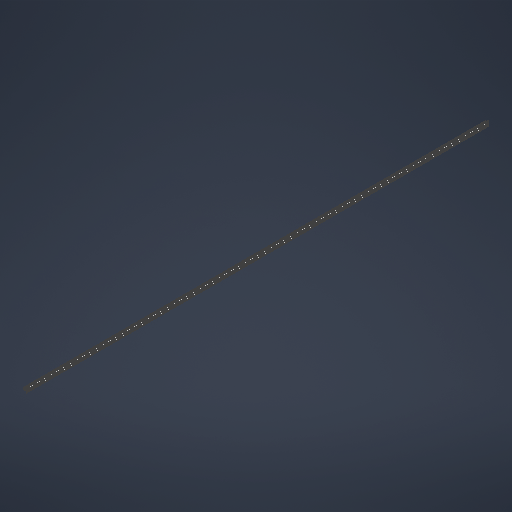
# Autodesk Inventor part: PLANTILLA SP40-04A TRAVESAÑO CENTRAL
Saved by Autodesk Inventor 2025 (Build 290162000, 162)
## iProperties
Created: 2026-01-20
Part Number: PLANTILLA SP40-04A TRAVESAÑO CENTRAL
Material: Aluminio
Document SubType Name: Modeling
Designer: ROLANDO
Density: 2.7 g/cm^3
Appearance: Satinado
Author: ROLANDO
Autodesk Inventor part; units mm, degrees
ref_plane "YZ Plane" through (0, 0, 0) normal (1, 0, 0) x (0, 1, 0)
ref_plane "XZ Plane" through (0, 0, 0) normal (0, 1, 0) x (-1, 0, 0)
ref_plane "XY Plane" through (0, 0, 0) normal (0, 0, 1) x (1, 0, 0)
sketch "Boceto1" plane through (0, 0, 0) normal (0, 0, 1) x (1, 0, 0)
  line L0 (-1.1139, -2.6665) -> (15.7105, -2.6665)
  line L1 (16.2861, -3.2421) -> (16.2861, -16.3665)
  line L2 (16.2861, -16.3665) -> (12.4861, -16.3665)
  line L3 (12.4861, -16.3665) -> (12.4861, -18.0065)
  line L4 (13.1802, -19.0165) -> (13.8861, -19.0165)
  line L5 (13.8861, -19.0165) -> (13.8861, -17.7665)
  line L6 (13.8861, -17.7665) -> (16.2861, -17.7665)
  line L7 (16.2861, -17.7665) -> (16.2861, -24.2665)
  line L8 (16.2861, -24.2665) -> (13.8861, -24.2665)
  line L9 (13.8861, -24.2665) -> (13.8861, -23.0165)
  line L10 (13.8861, -23.0165) -> (13.1802, -23.0165)
  line L11 (12.4861, -24.0265) -> (12.4861, -25.6665)
  line L12 (12.4861, -25.6665) -> (17.6861, -25.6665)
  line L13 (17.6861, -25.6665) -> (17.6861, 4.4835)
  line L14 (16.2861, -0.6909) -> (16.2861, 9.7335)
  line L15 (7.3361, 2.6189) -> (7.3361, -2.6665) construction
  arc A0 (6.2361, 3.2888) -> (8.4361, 3.2888) centre (7.3361, 1.3835) ccw
  line L16 (4.9491, 1.1335) -> (5.1503, 1.1335)
  line L17 (4.9491, 1.6335) -> (5.1503, 1.6335)
  line L18 (10.9772, -1.2665) -> (15.7105, -1.2665)
  line L19 (9.723, 1.1335) -> (9.5218, 1.1335)
  line L20 (9.723, 1.6335) -> (9.5218, 1.6335)
  line L21 (7.5861, -1.0034) -> (7.5861, -0.8022)
  line L22 (7.0861, -1.0034) -> (7.0861, -0.8022)
  arc A1 (7.0861, -1.0034) -> (7.5861, -1.0034) centre (7.3361, 1.3835) ccw
  arc A2 (9.723, 1.1335) -> (9.723, 1.6335) centre (7.3361, 1.3835) ccw
  arc A3 (4.9491, 1.6335) -> (4.9491, 1.1335) centre (7.3361, 1.3835) ccw
  circle A4 centre (7.3361, 1.3835) radius 2.4 construction
  line L23 (6.2361, 4.8271) -> (6.2361, 3.2888)
  line L24 (8.4361, 4.8271) -> (8.4361, 3.2888)
  arc A5 (10.4771, -0.406) -> (8.4361, 4.8271) centre (7.3361, 1.3835) ccw
  arc A6 (6.2361, 4.8271) -> (4.2085, -0.4294) centre (7.3361, 1.3835) ccw
  line L25 (12.4861, -18.0065) -> (13.1802, -19.0165)
  line L26 (12.4861, -24.0265) -> (13.1802, -23.0165)
  arc A7 (15.7105, -1.2665) -> (16.2861, -0.6909) centre (15.7105, -0.6909) ccw
  arc A8 (16.2861, -3.2421) -> (15.7105, -2.6665) centre (15.7105, -3.2421) ccw
  arc A9 (3.8851, -1.2665) -> (4.2085, -0.4294) centre (3.7105, -0.718) ccw
  arc A10 (10.4771, -0.406) -> (10.9772, -1.2665) centre (10.9772, -0.6909) ccw
  line L27 (-26.537, 4.4835) -> (21.9694, 4.4835) construction
  line L28 (-1.6139, -3.1665) -> (-1.6139, -7.0665)
  line L29 (-1.6139, -7.0665) -> (-4.0139, -7.0665)
  line L30 (-5.0139, -5.6665) -> (-3.5139, -5.6665)
  line L31 (-3.0139, -5.1665) -> (-3.0139, -3.1665)
  line L32 (-3.5139, -2.6665) -> (-20.7139, -2.6665)
  line L33 (-21.2139, -3.1665) -> (-21.2139, -5.1665)
  line L34 (-20.7139, -5.6665) -> (-19.2139, -5.6665)
  line L35 (-20.2139, -7.0665) -> (-22.6139, -7.0665)
  line L36 (3.8851, -1.2665) -> (-20.7139, -1.2665)
  line L37 (-21.2139, -0.7665) -> (-21.2139, 4.4835)
  line L38 (-22.6139, -7.0665) -> (-22.6139, 4.4835)
  line L39 (-19.2139, -5.6665) -> (-19.2139, -6.2653)
  line L40 (-19.2139, -6.2653) -> (-20.2139, -7.0665)
  line L41 (-5.0139, -5.6665) -> (-5.0139, -6.2653)
  line L42 (-5.0139, -6.2653) -> (-4.0139, -7.0665)
  line L43 (4.3997, 1.3835) -> (10.1666, 1.3835) construction
  arc A11 (-1.1139, -2.6665) -> (-1.6139, -3.1665) centre (-1.1139, -3.1665) ccw
  arc A12 (-3.0139, -3.1665) -> (-3.5139, -2.6665) centre (-3.5139, -3.1665) ccw
  arc A13 (-3.5139, -5.6665) -> (-3.0139, -5.1665) centre (-3.5139, -5.1665) ccw
  arc A14 (-20.7139, -2.6665) -> (-21.2139, -3.1665) centre (-20.7139, -3.1665) ccw
  arc A15 (-21.2139, -5.1665) -> (-20.7139, -5.6665) centre (-20.7139, -5.1665) ccw
  arc A16 (-21.2139, -0.7665) -> (-20.7139, -1.2665) centre (-20.7139, -0.7665) ccw
  line L44 (-1.1139, 11.6335) -> (15.7105, 11.6335)
  line L45 (16.2861, 12.2091) -> (16.2861, 25.3335)
  line L46 (16.2861, 25.3335) -> (12.4861, 25.3335)
  line L47 (12.4861, 25.3335) -> (12.4861, 26.9735)
  line L48 (13.1802, 27.9835) -> (13.8861, 27.9835)
  line L49 (13.8861, 27.9835) -> (13.8861, 26.7335)
  line L50 (13.8861, 26.7335) -> (16.2861, 26.7335)
  line L51 (16.2861, 26.7335) -> (16.2861, 33.2335)
  line L52 (16.2861, 33.2335) -> (13.8861, 33.2335)
  line L53 (13.8861, 33.2335) -> (13.8861, 31.9835)
  line L54 (13.8861, 31.9835) -> (13.1802, 31.9835)
  line L55 (12.4861, 32.9935) -> (12.4861, 34.6335)
  line L56 (12.4861, 34.6335) -> (17.6861, 34.6335)
  line L57 (17.6861, 34.6335) -> (17.6861, 4.4835)
  line L58 (12.4861, 26.9735) -> (13.1802, 27.9835)
  line L59 (12.4861, 32.9935) -> (13.1802, 31.9835)
  arc A17 (15.7105, 11.6335) -> (16.2861, 12.2091) centre (15.7105, 12.2091) ccw
  line L60 (-1.6139, 12.1335) -> (-1.6139, 16.0335)
  line L61 (-1.6139, 16.0335) -> (-4.0139, 16.0335)
  line L62 (-5.0139, 14.6335) -> (-3.5139, 14.6335)
  line L63 (-3.0139, 14.1335) -> (-3.0139, 12.1335)
  line L64 (-3.5139, 11.6335) -> (-20.7139, 11.6335)
  line L65 (-21.2139, 12.1335) -> (-21.2139, 14.1335)
  line L66 (-20.7139, 14.6335) -> (-19.2139, 14.6335)
  line L67 (-20.2139, 16.0335) -> (-22.6139, 16.0335)
  line L68 (15.7861, 10.2335) -> (-20.7139, 10.2335)
  line L69 (-21.2139, 9.7335) -> (-21.2139, 4.4835)
  line L70 (-22.6139, 16.0335) -> (-22.6139, 4.4835)
  line L71 (-19.2139, 14.6335) -> (-19.2139, 15.2323)
  line L72 (-19.2139, 15.2323) -> (-20.2139, 16.0335)
  line L73 (-5.0139, 14.6335) -> (-5.0139, 15.2323)
  line L74 (-5.0139, 15.2323) -> (-4.0139, 16.0335)
  arc A18 (-1.6139, 12.1335) -> (-1.1139, 11.6335) centre (-1.1139, 12.1335) ccw
  arc A19 (-3.5139, 11.6335) -> (-3.0139, 12.1335) centre (-3.5139, 12.1335) ccw
  arc A20 (-3.0139, 14.1335) -> (-3.5139, 14.6335) centre (-3.5139, 14.1335) ccw
  arc A21 (-21.2139, 12.1335) -> (-20.7139, 11.6335) centre (-20.7139, 12.1335) ccw
  arc A22 (-20.7139, 14.6335) -> (-21.2139, 14.1335) centre (-20.7139, 14.1335) ccw
  arc A23 (-20.7139, 10.2335) -> (-21.2139, 9.7335) centre (-20.7139, 9.7335) ccw
  arc A24 (16.2861, 9.7335) -> (15.7861, 10.2335) centre (15.7861, 9.7335) ccw
  point P0 (4.8546, -1.2453)
  point P1 (9.7949, -1.2665)
  point P2 (7.2983, -2.6665)
  point P3 (16.2861, -21.0165)
  point P4 (5.0497, 1.6335)
  point P5 (9.6224, 1.6335)
  point P6 (16.2861, 29.9835)
  dimension "d4" = 1.4
  dimension "d5" = 1.4
  dimension "d6" = 1.4
  dimension "d7" = 1.4
  dimension "d8" = 1.4
  dimension "d9" = 1.4
  dimension "d12" = 4.4
  dimension "d19" = 0.5
  dimension "d22" = 4.05
  dimension "d26" = 0.5
  dimension "d30" = 0.5
  dimension "d32" = 4.8
  dimension "d35" = 1.1
  dimension "d36" = 2.2
  dimension "d37" = 1.415
  dimension "d38" = 1.415
  dimension "d39" = 0.2
  dimension "d40" = 0.2
  dimension "d43" = 23
  dimension "d44" = 4
  dimension "d45" = 9.3
  dimension "d46" = 6.5
  dimension "d50" = 5.2
  dimension "d53" = 0.2
  dimension "d55" = 0.2
  dimension "d56" = 0.25
  dimension "d57" = 0.2
  dimension "d58" = 1.4
  dimension "d66" = 2
  dimension "d67" = 2
  dimension "d68" = 2.4
  dimension "d69" = 3.01
  dimension "d70" = 6.02
  dimension "d71" = 34.5
  dimension "d72" = 111
  dimension "d74" = 0.7058
  dimension "d75" = 0.7058
  dimension "d90" = 30.15
  dimension "d91" = 1.4
  dimension "d92" = 1.4
  dimension "d93" = 1.4
  dimension "d94" = 1.4
  dimension "d96" = 3
  dimension "d97" = 14.2
  dimension "d98" = 18.2
  dimension "d99" = 21
  dimension "d100" = 40.3
  dimension "d101" = 10.35
  dimension "d102" = 0.25
  dimension "d103" = 0.25
  dimension "d105" = 3.4
  dimension "d106" = 3.4
  dimension "d107" = 1
  dimension "d108" = 38.7
  dimension "d109" = 38.7
  dimension "d118" = 0.5
  dimension "d143" = 0.5
  dimension "d144" = 60.3
  dimension "d145" = 14.3
  dimension "d146" = 23.1
  dimension "d147" = 11.5
  dimension "d148" = 0.5756
  dimension "d149" = 1.4
  dimension "d150" = 4.2833
  constraints: 150 end point, 56 point on circle, 44 symmetric about line, 25 centre point, 21 tangent, 17 perpendicular, 13 point on line, 8 equal radius, 7 parallel, 6 collinear, 6 horizontal, 6 vertical, 4 midpoint, 3 coincident, 2 equal length, 7 other
  measures "d4" distance between parallel lines of L13 L1
  measures "d5" distance between parallel lines of L13 L7
  measures "d6" distance between parallel lines of L12 L8
  measures "d7" distance between parallel lines of L2 L6
  measures "d8" distance between parallel lines of L3 L5
  measures "d9" distance between parallel lines of L11 L9
  measures "d12" diameter of A0
  measures "d19" distance between parallel lines of L16 L17
  measures "d22" distance from line of A5.centre L0
  measures "d26" distance between parallel lines of L19 L20
  measures "d30" distance between parallel lines of L22 L21
  measures "d32" diameter of A4
  measures "d35" distance between parallel lines of L15 L23
  measures "d36" distance between parallel lines of L24 L23
  measures "d37" radial gap between concentric circles of A0 A5
  measures "d38" radial gap between concentric circles of A6 A0
  measures "d39" radial gap between concentric circles of A4 A0
  measures "d40" radial gap between concentric circles of A4 A0
  measures "d43" distance between parallel lines of L12 L0
  measures "d44" distance between parallel lines of L10 L4
  measures "d45" distance between parallel lines of L12 L2
  measures "d46" distance between parallel lines of L8 L6
  measures "d50" distance between parallel lines of L13 L11
  measures "d53" radial gap between concentric circles of A0 A3
  measures "d55" radial gap between concentric circles of A1 A0
  measures "d56" distance between parallel lines of L21 L15
  measures "d57" radial gap between concentric circles of A2 A0
  measures "d58" distance between parallel lines of L0 L18
  measures "d66" distance from line of point (16.286, -21.017) L4
  measures "d67" distance from line of point (16.286, -21.017) L10
  measures "d68" distance between parallel lines of L7 L5
  measures "d69" vertical distance of point (16.286, -21.017) L3.end
  measures "d70" distance of L3.end L11.start
  measures "d71" angle of L5 L25
  measures "d72" angle of L26 L25
  measures "d74" distance of L4.start L4.end
  measures "d75" distance of L9.end L10.end
  measures "d90" distance between parallel lines of L12 L27
  measures "d91" distance between parallel lines of L38 L37
  measures "d92" distance between parallel lines of L32 L36
  measures "d93" distance between parallel lines of L28 L31
  measures "d94" distance between parallel lines of L29 L30
  measures "d96" distance between parallel lines of L30 L32
  measures "d97" distance between parallel lines of L41 L39
  measures "d98" distance between parallel lines of L31 L33
  measures "d99" distance between parallel lines of L38 L28
  measures "d100" distance between parallel lines of L13 L38
  measures "d101" distance from line of L13 A0.centre
  measures "d102" distance from line of point (5.05, 1.633) L43
  measures "d103" distance from line of point (9.622, 1.633) L43
  measures "d105" distance between parallel lines of L28 L41
  measures "d106" distance between parallel lines of L39 L38
  measures "d107" horizontal distance of L41.end L29.end
  measures "d108" angle of L29 L42
  measures "d109" angle of L35 L40
  measures "d118" radius of A11
  measures "d143" radius of A24
  measures "d144" distance between parallel lines of L12 L56
  measures "d145" distance between parallel lines of L32 L64
  measures "d146" distance between parallel lines of L67 L35
  measures "d147" distance between parallel lines of L36 L68
  measures "d148" radius of A17
  measures "d149" distance between parallel lines of L1 L13
  measures "d150" distance from line of L27.end L13
extrude "Extrusión1" add sketch "Boceto1" against normal blind 5800
